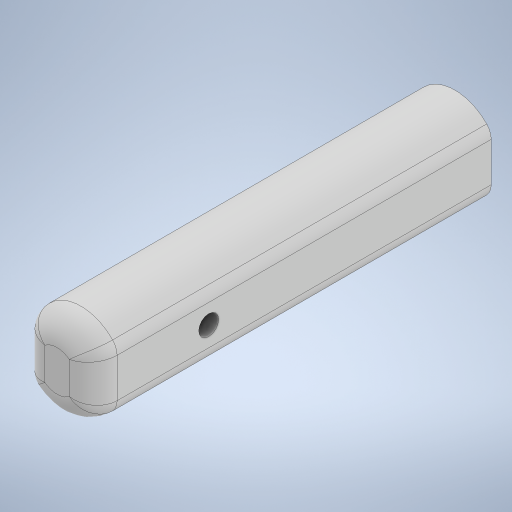
# Autodesk Inventor part: leg
Saved by Autodesk Inventor 2023 (Build 270158000, 158)
## iProperties
Created: 2023-11-07
Part Number: leg
Material: 一般
Document SubType Name: Modeling
Designer: bonju
Density: 1 g/cm^3
Appearance: 既定
Author: bonju
Autodesk Inventor part; units mm, degrees
ref_plane "YZ Plane" through (0, 0, 0) normal (1, 0, 0) x (0, 1, 0)
ref_plane "XZ Plane" through (0, 0, 0) normal (0, 1, 0) x (-1, 0, 0)
ref_plane "XY Plane" through (0, 0, 0) normal (0, 0, 1) x (1, 0, 0)
sketch "スケッチ1" plane through (0, 0, 0) normal (0, 0, 1) x (1, 0, 0)
  circle A0 centre (0, 0) radius 2.55
  line L0 (0, -7.77) -> (0, 7.77) projected
  arc A1 (-4.55, -3.178) -> (4.55, -3.178) centre (0, 0) ccw
  arc A2 (4.55, 3.178) -> (-4.55, 3.178) centre (0, 0) ccw
  line L1 (-4.55, -3.178) -> (-4.55, 3.178)
  line L2 (4.55, -3.178) -> (4.55, 3.178)
  dimension "d0" = 5.1
  dimension "d13" = 3
  dimension "d14" = 3
  dimension "d15" = 2
  constraints: 4 end point, 4 point on circle, 3 centre point, 2 symmetric about line, 1 coincident, 1 parallel, 1 vertical
  measures "d0" diameter of A0
  measures "d13" radial gap between concentric circles of A0 A1
  measures "d14" radial gap between concentric circles of A2 A0
  measures "d15" distance edge to line of A0 L1
extrude "押し出し1" add sketch "スケッチ1" along normal blind 50
sketch "スケッチ2" plane through (0, 0, 0) normal (0, 0, -1) x (-1, 0, 0)
  circle A0 centre (0, 0) radius 2.55
  dimension "d4" = 5.1
  constraints: 1 centre point, 1 coincident
  measures "d4" diameter of A0
extrude "押し出し2" cut sketch "スケッチ2" against normal blind 5.1
sketch "スケッチ4" plane through (-4.55, -3.178, 0) normal (-1, 0, 0) x (0, 0, 1)
  circle A0 centre (35.5, 3.178) radius 1.25
  line L0 (50, 6.3561) -> (50, 0) projected
  point P0 (0, 3.178)
  dimension "d16" = 2.5
  dimension "d17" = 14.5
  constraints: 1 centre point
  measures "d16" diameter of A0
  measures "d17" distance from line of L0 A0.centre
extrude "押し出し4" cut sketch "スケッチ4" along normal through all both and the other way through all
fillet "フィレット1" radius 3 4 edges at (0, -5.55, 50) (0, 5.55, 50) (-4.55, 0, 50) (4.55, 0, 50)
fillet "フィレット2" radius 2 12 edges at (4.0515, -3.0171, 48.6561) (2.1765, -2.3137, 49.9338) (4.55, -3.178, 23.5) (2.1765, 2.3137, 49.9338) (4.0515, 3.0171, 48.656) (4.55, 3.178, 23.5) (-2.1765, -2.3137, 49.9338) (-4.0515, -3.0171, 48.6561) (-4.55, -3.178, 23.5) (-4.0515, 3.0171, 48.656) (-2.1765, 2.3137, 49.9338) (-4.55, 3.178, 23.5)
